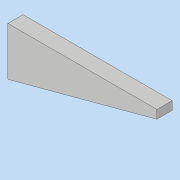
# Autodesk Inventor part: RudderStabilizingLowerFins
Saved by Autodesk Inventor 2017 (Build 210142000, 142)
## iProperties
Created: 2016-10-10
Part Number: RudderStabilizingLowerFins
Material: Generic
Document SubType Name: Modeling
Designer: techn
Density: 1 g/cm^3
Appearance: Default
Author: techn
Autodesk Inventor part; units mm, degrees
ref_plane "YZ Plane" through (0, 0, 0) normal (1, 0, 0) x (0, 1, 0)
ref_plane "XZ Plane" through (0, 0, 0) normal (0, 1, 0) x (-1, 0, 0)
ref_plane "XY Plane" through (0, 0, 0) normal (0, 0, 1) x (1, 0, 0)
sketch "Sketch1" plane through (0, 0, 0) normal (0, 0, 1) x (1, 0, 0)
  line L0 (0, 0) -> (31.163, 0)
  line L1 (31.163, 0) -> (31.163, -1.7663)
  line L2 (31.163, -1.7663) -> (0, -1.7663)
  line L3 (0, -1.7663) -> (0, 0)
  line L4 (0, -1.7663) -> (0, -10.1164)
  line L5 (0, -10.1164) -> (31.163, -1.7663)
  dimension "d0" = 31.163
  dimension "d1" = 10.1164
  dimension "d2" = 8.3501
  constraints: 12 end point, 2 parallel, 1 horizontal, 1 perpendicular, 1 vertical
  measures "d0" distance of L0.start L0.end
  measures "d1" distance of L0.start L4.end
  measures "d2" distance from line of L4.end L2
extrude "Extrusion1" add sketch "Sketch1" along normal blind 3.175
body "Solid1"
